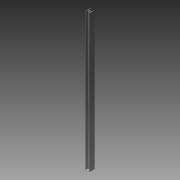
# Autodesk Inventor part: Bridge
Saved by Autodesk Inventor 2015 (Build 190159000, 159)
## iProperties
Created: 2016-12-02
Part Number: Bridge
Material: Generic
Document SubType Name: Modeling
Designer: Ernest
Density: 1 g/cm^3
Appearance: Default
Author: Ernest
Autodesk Inventor part; units mm, degrees
ref_plane "YZ Plane" through (0, 0, 0) normal (1, 0, 0) x (0, 1, 0)
ref_plane "XZ Plane" through (0, 0, 0) normal (0, 1, 0) x (-1, 0, 0)
ref_plane "XY Plane" through (0, 0, 0) normal (0, 0, 1) x (1, 0, 0)
sketch "Sketch1" plane through (0, 0, 0) normal (0, 0, 1) x (1, 0, 0)
  line L0 (0, 0) -> (3, 0)
  line L1 (3, 0) -> (3, 50)
  line L2 (3, 50) -> (0, 50)
  line L3 (0, 50) -> (0, 0)
  line L4 (3, 26.5) -> (37, 26.5)
  line L5 (37, 26.5) -> (37, 23.5)
  line L6 (37, 23.5) -> (3, 23.5)
  line L7 (3, 23.5) -> (3, 26.5)
  line L8 (37, 50) -> (40, 50)
  line L9 (40, 50) -> (40, 0)
  line L10 (40, 0) -> (37, 0)
  line L11 (37, 0) -> (37, 50)
  line L12 (0, 25) -> (40, 25) construction
  dimension "d3" = 3
  dimension "d4" = 40
  dimension "d9" = 1.5
  dimension "d10" = 50
  dimension "d11" = 25
  constraints: 26 end point, 6 parallel, 4 perpendicular, 4 point on line, 3 horizontal, 2 equal length, 2 midpoint
  measures "d3" distance of L1.end L2.end
  measures "d4" distance of L12.start L12.end
  measures "d9" distance between parallel lines of L12 L4
  measures "d10" distance of L8.end L9.end
  measures "d11" distance between parallel lines of L8 L12
extrude "Extrusion1" add sketch "Sketch1" along normal blind 1337.4
fillet "Fillet1" radius 0.75 4 edges at (3, 23.5, 668.7) (37, 23.5, 668.7) (37, 26.5, 668.7) (3, 26.5, 668.7)
body "Solid1"
